Autodesk Inventor part; units mm, degrees
(part 2 of 2)
  point P113 (-63.8301, 298.8246)
  point P114 (7.6927, 305.4688)
  point P115 (15.9625, 304.582)
  point P116 (23.93, 304.0598)
  point P117 (31.6358, 303.9236)
  point P118 (-16.2978, 305.1308)
  point P119 (-40.1878, 302.9114)
  point P120 (-305.1628, -15.6864)
  point P121 (-302.9913, -39.5808)
  point P122 (-220.8365, 127.5)
  point P123 (-305.4528, 8.3048)
  point P124 (-256.4356, 166.1662)
  point P125 (-210.5595, 221.4387)
  point P126 (-204.0848, 226.6592)
  point P127 (-198.0817, 231.9238)
  point P128 (-227.2843, 204.2358)
  point P129 (-242.6078, 185.7736)
  point P130 (-204.6908, -226.8746)
  point P131 (-186.2594, -242.2351)
  point P132 (-246.3111, -65.9989)
  point P133 (-221.8601, -210.1154)
  point P134 (-298.8246, -63.8301)
  point P135 (-305.4688, 7.6927)
  point P136 (-304.582, 15.9625)
  point P137 (-304.0598, 23.93)
  point P138 (-303.9236, 31.6358)
  point P139 (-305.1308, -16.2978)
  point P140 (-302.9114, -40.1878)
  dimension "d1" = 330
  dimension "d2" = 45
  dimension "d3" = 5
  dimension "d4" = 5
  dimension "d6" = 30
  dimension "d7" = 20
  dimension "d8" = 20
  dimension "d14" = 20
  dimension "d35" = 3
  dimension "d36" = 1.5
  dimension "d44" = 80
  dimension "d47" = 360
  dimension "d50" = 10
  dimension "d52" = 10
  dimension "d53" = 40
  dimension "d54" = 5
  dimension "d55" = 10
  dimension "d61" = 40
  dimension "d63" = 5
  dimension "d64" = 10
  dimension "d66" = 40
  dimension "d69" = 360
  constraints: 679 point on circle, 544 end point, 344 centre point, 106 coincident, 72 point on line, 9 midpoint, 9 symmetric about line, 4 parallel, 2 perpendicular, 2 tangent, 1 collinear, 1 vertical, 2218 other
  measures "d1" diameter of A1
  measures "d2" angle of L1 L0
  measures "d3" angle of L2 L0
  measures "d4" angle of L1 L3
  measures "d6" radial gap between concentric circles of A3 A1
  measures "d7" radial gap between concentric circles of A3 A4
  measures "d8" radial gap between concentric circles of A5 A2
  measures "d14" angle of L3 L8
  measures "d35" angle of L0 L9
  measures "d36" angle of L9 L10
  measures "d44" radius of A9
  measures "d50" radial gap between concentric circles of A90 A89
  measures "d52" angle of L11 L0
  measures "d53" distance of L12.start L12.end
  measures "d54" distance between parallel lines of L12 L14
  measures "d55" radial gap between concentric circles of A91 A1
  measures "d63" distance between parallel lines of L22 L20
  measures "d64" angle of L22 L8
extrude "Extrusion1" add sketch "Sketch2" along normal blind 5 contours L0 A8 L11 A89 | L5 L0 A4 L2 | A90 L11 L27 L28 L29 A4 L0 | A9 A0 A10 A8 | L11 A8 L3 A89 | A89 L3 A90 L11 | A4 L4 L2 | A90 L3 A4 L11 L29 L30 L27 | L3 A8 L1 A89 | A8 A168 A0 A169 | A1 L11 A91 L3 | A4 L11 A3 L0 | A170 A0 A171 A8 | A90 L1 L7 L3 | L0 A3 L11 A91 | A91 L3 A3 L1 | A91 L11 A3 L3 | A4 L3 A3 L11 | A154 A0 A155 A8 | A8 A156 A0 A157 | A166 A0 A167 A8 | A3 L6 L1 | A8 A158 A0 A159 | A164 A0 A165 A8 | A8 A160 A0 A161 | A162 A0 A163 A8
body "Solid1"
